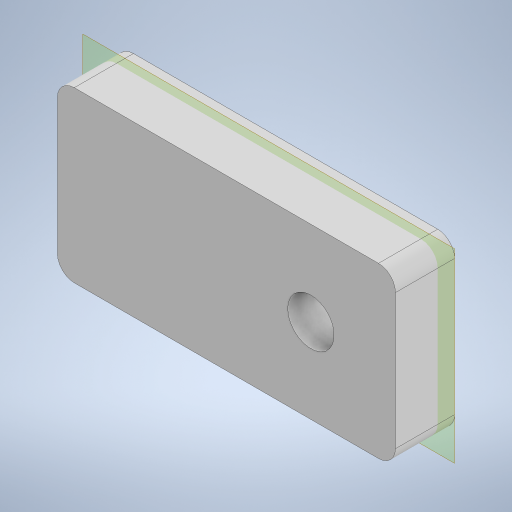
# Autodesk Inventor part: MagnetHolderV1
Saved by Autodesk Inventor 2024.4 (Build 284460000, 460)
## iProperties
Created: 2025-12-08
Part Number: MagnetHolderV1
Material: Generic
Document SubType Name: Modeling
Designer: jonas
Density: 1 g/cm^3
Appearance: Default
Author: jonas
Autodesk Inventor part; units mm, degrees
ref_plane "YZ Plane" through (0, 0, 0) normal (1, 0, 0) x (0, 1, 0)
ref_plane "XZ Plane" through (0, 0, 0) normal (0, 1, 0) x (-1, 0, 0)
ref_plane "XY Plane" through (0, 0, 0) normal (0, 0, 1) x (1, 0, 0)
sketch "Sketch1" plane through (0, 0, 0) normal (0, 1, 0) x (-1, 0, 0)
  line L0 (2.1258, 0) -> (-2.1258, 0) construction
  line L1 (0, 4.2515) -> (0, -4.2515) construction
  line L2 (20, 10) -> (-20, 10)
  line L3 (-20, 10) -> (-20, -10)
  line L4 (-20, -10) -> (20, -10)
  line L5 (20, -10) -> (20, 10)
  point P0 (0, 0)
  point P1 (0, 0)
  dimension "d1" = 20
  dimension "d2" = 20
  dimension "d3" = 20
  constraints: 12 end point, 2 horizontal, 2 midpoint, 2 parallel, 1 coincident, 1 perpendicular, 1 vertical, 1 other
  measures "d1" distance between parallel lines of L1 L5
  measures "d2" distance of L4.end L2.start
  measures "d3" distance from line of L1.end L3
extrude "Extrusion1" add sketch "Sketch1" along normal blind 7
sketch "Sketch2" plane through (0, 7, 0) normal (0, 1, 0) x (1, 0, 0)
  point P0 (0, 0)
  point P1 (10, 0)
  dimension "d6" = 10
  constraints: 1 horizontal alignment
  measures "d6" distance of point (0, 0) point (10, 0)
hole "Hole1" at (10, 7, 0) direction (0, -1, 0) diameter 5.5 end through all countersink diameter 10.4 countersink angle 90 clearance for "Countersunk Flat Head Screw DIN EN ISO 2009" size "M5" standard "DIN"
ref_plane "Work Plane1" through (0, 5, 0) normal (0, 1, 0) x (1, 0, 0)
sketch "Sketch3" plane through (0, 5, 0) normal (0, 1, 0) x (1, 0, 0)
  circle A0 centre (-8.9944, 0) radius 3
  point P0 (0, 0)
  dimension "d15" = 6
  constraints: 1 centre point
  measures "d15" diameter of A0
extrude "Extrusion2" cut sketch "Sketch3" against normal blind 1.7
fillet "Fillet1" radius 2 4 edges at (-20, 3.5, 10) (-20, 3.5, -10) (20, 3.5, 10) (20, 3.5, -10)
body "Solid1"
